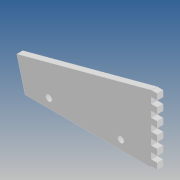
# Autodesk Inventor part: KB33-046-004-009 - Передняя левая боковая пластина
Saved by Autodesk Inventor 2020 (Build 240168000, 168)
## iProperties
Created: 2021-06-25
Part Number: KB33-046-004-009 - Передняя левая боковая пластина
Material: Типовые
Document SubType Name: Modeling
Designer: Петров Иван
Mass: 11.7793 g
Surface Area: 71.5428 cm^2
Volume: 11.7793 cm^3
Density: 1 g/cm^3
Appearance: По умолчанию
Author: Петров Иван
Autodesk Inventor part; units mm, degrees
ref_plane "YZ Plane" through (0, 0, 0) normal (1, 0, 0) x (0, 1, 0)
ref_plane "XZ Plane" through (0, 0, 0) normal (0, 1, 0) x (-1, 0, 0)
ref_plane "XY Plane" through (0, 0, 0) normal (0, 0, 1) x (1, 0, 0)
sketch "Эскиз1" plane through (0, 0, 0) normal (0, 0, 1) x (1, 0, 0)
  line L0 (-1.0718, 4) -> (83.0251, 4)
  circle A0 centre (14.7479, 10) radius 2
  circle A1 centre (62.7479, 10) radius 2
  line L1 (-1.0718, 4) -> (-3.896, 14.54)
  line L2 (83.0251, 4) -> (83.0251, 48.71)
  line L3 (-3.896, 14.54) -> (-6.6159, 24.6909)
  line L4 (-6.6159, 24.6909) -> (83.0251, 48.71)
  dimension "d0" = 10.509
  constraints: 10 end point, 2 centre point, 1 point on line
  measures "d0" distance of L1.end L3.end
extrude "Выдавливание1" add sketch "Эскиз1" along normal blind 4
sketch "Эскиз2" plane through (83.0251, 4, 0) normal (1, 0, 0) x (0, 0, -1)
  line L0 (-4, 0) -> (-4, 44.71) projected
  line L1 (0, 0) -> (0, 44.71) projected
  line L2 (-4, 44.71) -> (0, 44.71)
  line L3 (0, 44.71) -> (0, 40.71)
  line L4 (0, 40.71) -> (-4, 40.71)
  line L5 (-4, 40.71) -> (-4, 44.71)
  point P0 (0, -4)
  point P1 (-4, 40.71)
  dimension "d3" = 4
  constraints: 8 end point, 2 parallel, 1 horizontal, 1 perpendicular, 1 point on line
  measures "d3" distance of L2.end L3.end
extrude "Выдавливание2" add sketch "Эскиз2" along normal blind 4
pattern_linear "Прямоуг.массив1" count 6 spacing 8 along (0, -1, 0) of "Выдавливание2"
